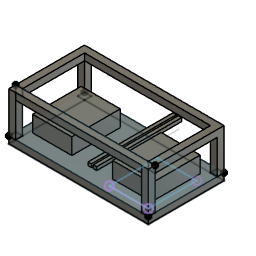
Gantry v4 (Autodesk Fusion 360 design; units mm, degrees)
Autodesk Fusion 360 part; units mm, degrees
sketch "Sketch1" plane through (0, 0, 0) normal (0, 1, 0) x (1, 0, 0)
  line L0 (-45.72, 30.48) -> (246.38, 30.48)
  line L1 (246.38, 30.48) -> (246.38, -331.47)
  line L2 (246.38, -331.47) -> (-45.72, -331.47)
  line L3 (-45.72, -331.47) -> (-45.72, 30.48)
  dimension "d1" = 292.1
  dimension "d2" = 361.95
  constraint horizontal L0
  constraint vertical L1
  constraint horizontal L2
  constraint vertical L3
  measures "d1" distance of L0.start L0.end
  measures "d2" distance of L0.start L2.end
extrude "Extrude1" add sketch "Sketch1" along normal blind 57.15 makes body 1
move_body "Move1" bodies 1 to x (1, 0, 0) y (0, 1, 0) z (0, 0, 1) at (0, 127, 0)
sketch "Sketch6" plane through (0, 0, 0) normal (0, 1, 0) x (1, 0, 0)
  line L0 (347.98, 132.08) -> (-693.42, 132.08)
  line L1 (-693.42, 132.08) -> (-693.42, -433.07)
  line L2 (-693.42, -433.07) -> (347.98, -433.07)
  line L3 (347.98, -433.07) -> (347.98, 132.08)
  line L4 (246.38, -331.47) -> (-45.72, -331.47)
  point P0 (246.38, -331.47)
  point P1 (246.38, 30.48)
  point P2 (-45.72, -331.47)
  dimension "d5" = 101.6
  dimension "d6" = 101.6
  dimension "d7" = 101.6
  dimension "d8" = 647.7
  dimension "d9" = 292.1
  constraint horizontal L0
  constraint vertical L1
  constraint horizontal L2
  constraint vertical L3
  measures "d5" distance of L2 P0
  measures "d6" distance of L0 P1
  measures "d7" distance of L3 P0
  measures "d8" distance of L1 P2
  measures "d9" distance of P0 P2
extrude "Extrude2" add sketch "Sketch6" along normal blind 50.8 separate body makes body 2
move_body "Move2" bodies 1 to x (1, 0, 0) y (0, 1, 0) z (0, 0, 1) at (0, 50.8, 0)
move_face "MoveFace1" by (0, 63.5, 0) 1 faces at (51.6467, 234.95, 210.82) on bodies 1
move_body "Move3" bodies 1 to x (1, 0, 0) y (0, 1, 0) z (0, 0, 1) at (0, 57.15, 0)
move_body "Move4" bodies 1 to x (1, 0, 0) y (0, 1, 0) z (0, 0, 1) at (0, -177.8, 0)
sketch "Sketch7" plane through (0, 50.8, 0) normal (0, 1, 0) x (-1, 0, 0)
  line L0 (-347.98, 433.07) -> (-347.98, -132.08)
  line L1 (-347.98, -132.08) -> (693.42, -132.08)
  line L2 (693.42, -132.08) -> (693.42, 433.07)
  line L3 (693.42, 433.07) -> (-347.98, 433.07)
  line L4 (-347.98, -132.08) -> (-297.18, -132.08)
  line L5 (-297.18, -132.08) -> (-297.18, -81.28)
  line L6 (-297.18, -81.28) -> (-347.98, -81.28)
  line L7 (-347.98, -81.28) -> (-347.98, -132.08)
  dimension "d12" = 50.8
  dimension "d13" = 50.8
  constraint horizontal L4
  constraint vertical L5
  constraint horizontal L6
  constraint vertical L7
  constraint coincident L0.end L1.start
  measures "d12" distance of L0.end L6.end
  measures "d13" distance of L0.end L4.end
extrude "Extrude3" add sketch "Sketch7" along normal blind 304.8 contours L0 L1 L4 L5 L6 L7 bodies 2
sketch "Sketch8" plane through (0, 50.8, 0) normal (0, 1, 0) x (-1, 0, 0)
  line L0 (-297.18, -81.28) -> (-297.18, -132.08)
  line L1 (-297.18, -132.08) -> (693.42, -132.08)
  line L2 (693.42, -132.08) -> (693.42, 433.07)
  line L3 (693.42, 433.07) -> (-347.98, 433.07)
  line L4 (-347.98, 433.07) -> (-347.98, -81.28)
  line L5 (-347.98, -81.28) -> (-297.18, -81.28)
  line L6 (-347.98, 433.07) -> (-297.18, 433.07)
  line L7 (-297.18, 433.07) -> (-297.18, 382.27)
  line L8 (-297.18, 382.27) -> (-347.98, 382.27)
  line L9 (-347.98, 382.27) -> (-347.98, 433.07)
  line L10 (693.42, 433.07) -> (642.62, 433.07)
  line L11 (642.62, 433.07) -> (642.62, 382.27)
  line L12 (642.62, 382.27) -> (693.42, 382.27)
  line L13 (693.42, 382.27) -> (693.42, 433.07)
  line L14 (693.42, -132.08) -> (642.62, -132.08)
  line L15 (642.62, -132.08) -> (642.62, -81.28)
  line L16 (642.62, -81.28) -> (693.42, -81.28)
  line L17 (693.42, -81.28) -> (693.42, -132.08)
  dimension "d16" = 50.8
  dimension "d17" = 50.8
  dimension "d18" = 50.8
  dimension "d19" = 50.8
  dimension "d20" = 50.8
  dimension "d21" = 50.8
  constraint horizontal L6
  constraint vertical L7
  constraint horizontal L8
  constraint vertical L9
  constraint coincident L3.end L4.start
  constraint horizontal L10
  constraint vertical L11
  constraint horizontal L12
  constraint vertical L13
  constraint coincident L2.end L3.start
  constraint horizontal L14
  constraint vertical L15
  constraint horizontal L16
  constraint vertical L17
  constraint coincident L1.end L2.start
  measures "d16" distance of L3.end L8.end
  measures "d17" distance of L3.end L6.end
  measures "d18" distance of L2.end L10.end
  measures "d19" distance of L2.end L12.end
  measures "d20" distance of L1.end L14.end
  measures "d21" distance of L1.end L16.end
extrude "Extrude4" add sketch "Sketch8" along normal blind 304.8 contours L1 L2 L14 L15 L16 L17 bodies 2
sketch "Sketch9" plane through (0, 50.8, 0) normal (0, 1, 0) x (-1, 0, 0)
extrude "Extrude5" add sketch "Sketch8" along normal blind 304.8 contours L3 L4 L6 L7 L8 L9 bodies 2
extrude "Extrude6" add sketch "Sketch8" along normal blind 304.8 contours L2 L3 L10 L11 L12 L13 bodies 2
sketch "Sketch10" plane through (-642.62, 0, 0) normal (1, 0, 0) x (0, 0, -1)
  line L0 (-433.07, 50.8) -> (-382.27, 50.8)
  line L1 (-382.27, 50.8) -> (-382.27, 355.6)
  line L2 (-382.27, 355.6) -> (-433.07, 355.6)
  line L3 (-433.07, 355.6) -> (-433.07, 50.8)
  line L4 (-431.8, 355.6) -> (-381, 355.6)
  line L5 (-381, 355.6) -> (-381, 304.8)
  line L6 (-381, 304.8) -> (-431.8, 304.8)
  line L7 (-431.8, 304.8) -> (-431.8, 355.6)
  dimension "d28" = 50.8
  dimension "d29" = 50.8
  constraint horizontal L4
  constraint vertical L5
  constraint horizontal L6
  constraint vertical L7
  constraint coincident L2 L4.start
  measures "d28" distance of L4.start L4.end
  measures "d29" distance of L4.start L6.end
extrude "Extrude7" add sketch "Sketch10" along normal blind 939.8 contours L1 L2 L4 L6 L7 bodies 2
sketch "Sketch11" plane through (-642.62, 0, 0) normal (1, 0, 0) x (0, 0, -1)
  line L0 (81.28, 50.8) -> (132.08, 50.8)
  line L1 (132.08, 50.8) -> (132.08, 355.6)
  line L2 (132.08, 355.6) -> (81.28, 355.6)
  line L3 (81.28, 355.6) -> (81.28, 50.8)
  line L4 (81.28, 355.6) -> (132.08, 355.6)
  line L5 (132.08, 355.6) -> (132.08, 304.8)
  line L6 (132.08, 304.8) -> (81.28, 304.8)
  line L7 (81.28, 304.8) -> (81.28, 355.6)
  dimension "d32" = 50.8
  dimension "d33" = 50.8
  constraint horizontal L4
  constraint vertical L5
  constraint horizontal L6
  constraint vertical L7
  constraint coincident L2.end L3.start
  measures "d32" distance of L2.end L1.end
  measures "d33" distance of L2.end L6.end
extrude "Extrude8" add sketch "Sketch11" along normal blind 939.8 contours L1 L2 L3 L4 L5 L6 L7 bodies 2
sketch "Sketch12" plane through (0, 0, 382.27) normal (0, 0, -1) x (-1, 0, 0)
  line L0 (642.62, 50.8) -> (693.42, 50.8)
  line L1 (693.42, 50.8) -> (693.42, 355.6)
  line L2 (693.42, 355.6) -> (642.62, 355.6)
  line L3 (642.62, 355.6) -> (-297.18, 355.6)
  line L4 (-297.18, 355.6) -> (-347.98, 355.6)
  line L5 (-347.98, 355.6) -> (-347.98, 50.8)
  line L6 (-347.98, 50.8) -> (-297.18, 50.8)
  line L7 (-297.18, 50.8) -> (-297.18, 304.8)
  line L8 (-297.18, 304.8) -> (642.62, 304.8)
  line L9 (642.62, 304.8) -> (642.62, 50.8)
  line L10 (-347.98, 355.6) -> (-297.18, 355.6)
  line L11 (-297.18, 355.6) -> (-297.18, 304.8)
  line L12 (-297.18, 304.8) -> (-347.98, 304.8)
  line L13 (-347.98, 304.8) -> (-347.98, 355.6)
  line L14 (693.42, 355.6) -> (642.62, 355.6)
  line L15 (642.62, 355.6) -> (642.62, 304.8)
  line L16 (642.62, 304.8) -> (693.42, 304.8)
  line L17 (693.42, 304.8) -> (693.42, 355.6)
  dimension "d36" = 50.8
  dimension "d37" = 50.8
  dimension "d38" = 50.8
  dimension "d39" = 50.8
  constraint horizontal L10
  constraint vertical L11
  constraint horizontal L12
  constraint vertical L13
  constraint coincident L4.end L5.start
  constraint horizontal L14
  constraint vertical L15
  constraint horizontal L16
  constraint vertical L17
  constraint coincident L1.end L2.start
  measures "d36" distance of L4.end L3.end
  measures "d37" distance of L4.end L12.end
  measures "d38" distance of L1.end L2.end
  measures "d39" distance of L1.end L16.end
extrude "Extrude9" add sketch "Sketch12" along normal blind 463.55 contours L4 L5 L10 L11 L12 L13 bodies 2
extrude "Extrude10" add sketch "Sketch12" along normal blind 463.55 contours L1 L2 L14 L15 L16 L17 bodies 2
sketch "Sketch13" plane through (0, 50.8, 0) normal (0, 1, 0) x (-1, 0, 0)
copy_body "CopyPasteBodies1" bodies 1 makes body 3
move_body "Move5" bodies 3 to x (1, 0, 0) y (0, 1, 0) z (0, 0, 1) at (-558.8, 0, 0)
sketch "Sketch14" plane through (0, 50.8, 0) normal (0, 1, 0) x (-1, 0, 0)
move_body "Move6" bodies 3 to x (1, 0, 0) y (0, 1, 0) z (0, 0, 1) at (-38.1, 0, 0)
move_body "Move7" bodies 3 to x (1, 0, 0) y (0, 1, 0) z (0, 0, 1) at (25.4, 0, 0)
move_body "Move8" bodies 1 to x (1, 0, 0) y (0, 1, 0) z (0, 0, 1) at (25.4, 0, 0)
sketch "Sketch15" plane through (0, 50.8, 0) normal (0, 1, 0) x (-1, 0, 0)
  line L0 (140.97, 330.2) -> (166.37, 330.2)
  line L1 (166.37, 330.2) -> (166.37, -304.8)
  line L2 (166.37, -304.8) -> (140.97, -304.8)
  line L3 (140.97, -304.8) -> (140.97, 330.2)
  line L4 (179.07, 330.2) -> (204.47, 330.2)
  line L5 (204.47, 330.2) -> (204.47, -304.8)
  line L6 (204.47, -304.8) -> (179.07, -304.8)
  line L7 (179.07, -304.8) -> (179.07, 330.2)
  point P0 (20.32, 331.47)
  point P1 (325.12, 331.47)
  dimension "d53" = 304.8
  dimension "d54" = 25.4
  dimension "d55" = 635
  dimension "d56" = 120.65
  dimension "d57" = 25.4
  dimension "d58" = 635
  dimension "d59" = 12.7
  constraint horizontal L0
  constraint vertical L1
  constraint horizontal L2
  constraint vertical L3
  constraint horizontal L4
  constraint vertical L5
  constraint horizontal L6
  constraint vertical L7
  measures "d53" distance of P0 P1
  measures "d54" distance of L0.start L0.end
  measures "d55" distance of L0.start L2.end
  measures "d56" horizontal distance of P0 L0.start
  measures "d57" distance of L4.start L4.end
  measures "d58" distance of L4.start L6.end
  measures "d59" distance of L1 L7
extrude "Extrude11" add sketch "Sketch15" along normal blind 25.4 bodies 2
